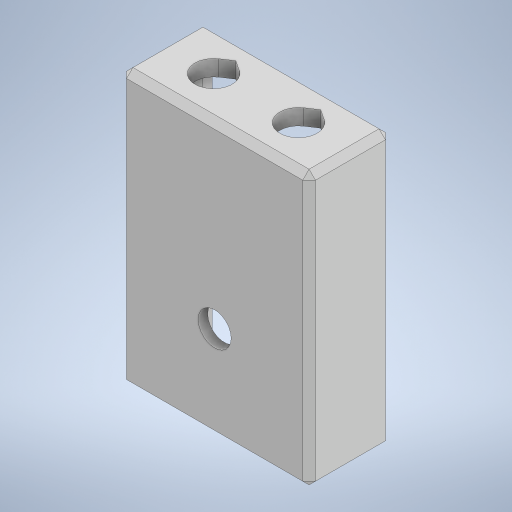
# Autodesk Inventor part: PotiBoxCase
Saved by Autodesk Inventor 2024.3 (Build 283343000, 343)
## iProperties
Created: 2025-03-30
Part Number: PotiBoxCase
Material: Generisch
Document SubType Name: Modeling
Designer: maxho
Density: 1 g/cm^3
Appearance: Vorgabe
Author: maxho
## iProperties of the stored document PotiBoxCase_3D-Druck.ipt
Created: 2025-03-30
Part Number: PotiBoxCase_3D-Druck
Material: Generisch
Document SubType Name: Modeling
Designer: maxho
Density: 1 g/cm^3
Appearance: Vorgabe
Author: maxho
Autodesk Inventor part; units mm, degrees
ref_plane "YZ Plane" through (0, 0, 0) normal (1, 0, 0) x (0, 1, 0)
ref_plane "XZ Plane" through (0, 0, 0) normal (0, 1, 0) x (-1, 0, 0)
ref_plane "XY Plane" through (0, 0, 0) normal (0, 0, 1) x (1, 0, 0)
sketch "Skizze1" plane through (0, 0, 0) normal (0, 1, 0) x (-1, 0, 0)
  line L0 (-29.7, -43) -> (29.7, -43)
  line L1 (29.7, -43) -> (29.7, 43)
  line L2 (29.7, 43) -> (-29.7, 43)
  line L3 (-29.7, 43) -> (-29.7, -43)
  line L4 (-29.7, -43) -> (29.7, 43) construction
  line L5 (29.7, -43) -> (-29.7, 43) construction
  point P0 (0, 0)
  dimension "d2" = 59.4
  dimension "d3" = 86
  constraints: 12 end point, 2 midpoint, 2 parallel, 1 horizontal, 1 perpendicular
  measures "d2" distance of L1.end L2.end
  measures "d3" distance of L0.end L1.end
extrude "Extrusion1" add sketch "Skizze1" along normal blind 26
shell "Wandung1" thickness 3 removed faces 1 at (-9.9, 26, -14.3333)
sketch "Skizze2" plane through (-29.7, 0, 43) normal (0, 0, 1) x (1, 0, 0)
  line L0 (0, 0) -> (59.4, 0) construction
  line L1 (59.4, 0) -> (59.4, 26) construction
  line L2 (0, 26) -> (59.4, 26) construction
  line L3 (0, 0) -> (0, 26) construction
  line L4 (3, 3) -> (56.4, 3) construction
  line L5 (3, 3) -> (3, 26) construction
  line L6 (56.4, 26) -> (3, 26) construction
  line L7 (56.4, 3) -> (56.4, 26) construction
  circle A0 centre (16.35, 13) radius 5.85
  circle A1 centre (43.05, 13) radius 5.85
  line L8 (3, 23) -> (56.4, 23) construction
  line L9 (3, 23) -> (29.7, 3) construction
  line L10 (29.7, 3) -> (56.4, 23) construction
  line L11 (19.5626, 17.8889) -> (16.35, 20)
  line L12 (16.35, 20) -> (13.1374, 17.8889)
  line L13 (46.2626, 17.8889) -> (43.05, 20)
  line L14 (43.05, 20) -> (39.8374, 17.8889)
  point P0 (29.7, 0)
  dimension "d5" = 11.7
  dimension "d19" = 3
  dimension "d20" = 7
  constraints: 14 end point, 4 point on circle, 4 tangent, 3 midpoint, 2 centre point, 2 point on line, 2 vertical alignment, 1 equal radius, 1 horizontal alignment, 1 perpendicular
  measures "d5" diameter of A0
  measures "d19" distance between parallel lines of L2 L8
  measures "d20" distance of A0.centre L11.end
extrude "Extrusion2" cut sketch "Skizze2" against normal up to surface (3 mm away)
sketch "Skizze3" plane through (0, 0, 0) normal (0, -1, 0) x (1, 0, 0)
  line L0 (-29.7, -43) -> (-29.7, 43) construction
  line L1 (29.7, -43) -> (-29.7, -43) construction
  line L2 (29.7, 43) -> (29.7, -43) construction
  line L3 (-29.7, 43) -> (29.7, 43) construction
  line L4 (-26.7, -40) -> (-26.7, 40) construction
  line L5 (-26.7, 40) -> (26.7, 40) construction
  line L6 (26.7, 40) -> (26.7, -40) construction
  line L7 (26.7, -40) -> (-26.7, -40) construction
  circle A0 centre (0, -13.3333) radius 5.205
  line L8 (0, -40) -> (0, -13.3333) construction
  line L9 (0, -13.3333) -> (0, 13.3333) construction
  line L10 (0, 13.3333) -> (0, 40) construction
  point P0 (0, 0)
  dimension "d8" = 10.41
  constraints: 6 end point, 2 collinear, 2 midpoint, 1 centre point, 1 point on line, 1 vertical
  measures "d8" diameter of A0
extrude "Extrusion3" cut sketch "Skizze3" against normal through all
sketch "Skizze4" plane through (29.7, 0, -43) normal (0, 0, -1) x (-1, 0, 0)
  line L0 (0, 0) -> (59.4, 0) construction
  line L1 (59.4, 0) -> (59.4, 26) construction
  line L2 (0, 26) -> (59.4, 26) construction
  line L3 (0, 0) -> (0, 26) construction
  line L4 (3, 3) -> (56.4, 3) construction
  line L5 (24.495, 3) -> (34.905, 3) construction
  line L6 (56.4, 3) -> (3, 3) construction
  line L7 (3, 3) -> (56.4, 3) construction
  line L8 (56.4, 3) -> (56.4, 26) construction
  line L9 (3, 3) -> (3, 26) construction
  line L10 (56.4, 26) -> (57.6426, 23) construction
  line L11 (57.6426, 23) -> (1.7574, 23) construction
  line L12 (1.7574, 23) -> (3, 26) construction
  line L13 (56.5082, 26) -> (57.7923, 22.9)
  line L14 (57.7923, 22.9) -> (1.6077, 22.9)
  line L15 (1.6077, 22.9) -> (2.8918, 26)
  line L16 (2.8918, 26) -> (56.5082, 26)
  line L17 (59.4, 26) -> (0, 26) projected
  point P0 (29.7, 0)
  point P1 (29.7, 26)
  point P2 (29.7, 23)
  point P3 (29.7, 26)
  dimension "d11" = 3
  dimension "d12" = 22.5
  dimension "d13" = 0.1
  constraints: 14 end point, 4 midpoint, 1 collinear, 1 horizontal, 1 vertical alignment, 2 other
  measures "d11" distance between parallel lines of L2 L11
  measures "d12" angle of L10 L8
  measures "d13" distance between parallel lines of L10 L13
extrude "Extrusion4" cut sketch "Skizze4" against normal up to surface (83 mm away)
chamfer "Fasen1" distance 2 angle 45 13 edges at (-29.7, 13, -43) (-29.7, 0, 0) (0, 0, -43) (29.7, 13, -43) (29.7, 0, 0) (0, 0, 43) (-29.7, 13, 43) (29.7, 13, 43) (-29.7, 26, 0) (0, 26, 43) (29.7, 26, 0) (28.2541, 26, -43) (-28.2541, 26, -43)
sketch "Skizze5" plane through (26.7, 3, 40) normal (0, 0, -1) x (-1, 0, 0)
  line L0 (0, 0) -> (0, 19.9) projected
  line L1 (53.4, 0) -> (0, 0) projected
  line L2 (53.4, 0) -> (53.4, 19.9) projected
  line L3 (53.4, 19.9) -> (54.7923, 19.9) projected
  line L4 (54.7923, 19.9) -> (53.5082, 23) projected
  line L5 (-0.1082, 23) -> (53.5082, 23) projected
  line L6 (-0.1082, 23) -> (-1.3923, 19.9) projected
  line L7 (-1.3923, 19.9) -> (0, 19.9) projected
  arc A0 (10.1374, 14.8889) -> (16.5626, 14.8889) centre (13.35, 10) ccw projected
  line L8 (10.1374, 14.8889) -> (13.35, 17) projected
  line L9 (13.35, 17) -> (16.5626, 14.8889) projected
  line L10 (40.05, 17) -> (43.2626, 14.8889) projected
  arc A1 (36.8374, 14.8889) -> (43.2626, 14.8889) centre (40.05, 10) ccw projected
  line L11 (36.8374, 14.8889) -> (40.05, 17) projected
  line L12 (0, 19.9) -> (53.4, 19.9)
  point P0 (26.7, -3)
  constraints: 2 end point, 1 horizontal
extrude "Extrusion5" add sketch "Skizze5" along normal blind 2 contours L0 L12 L2 L1
sketch "Skizze6" plane through (-26.7, 3, -40) normal (0, 1, 0) x (1, 0, 0)
  line L0 (18.1388, -45.7075) -> (30.6952, -45.7075) construction
  line L1 (30.6952, -45.7075) -> (30.6952, -51.3198) construction
  line L2 (30.6952, -51.3198) -> (18.1388, -51.3198) construction
  line L3 (18.1388, -51.3198) -> (18.1388, -45.7075) construction
  line L4 (20.9099, -49.2784) -> (18.5983, -49.2784)
  line L5 (18.5983, -49.2784) -> (18.5983, -48.6686)
  line L6 (18.5983, -48.6686) -> (19.3357, -48.6686)
  line L7 (19.3357, -48.6686) -> (19.3357, -46.8165)
  line L8 (19.3357, -46.8165) -> (18.5983, -46.8165)
  line L9 (18.5983, -46.8165) -> (18.5983, -46.2464)
  spline S0 degree 2 poles (18.5983, -46.2464) (18.76, -46.2464) (19.0805, -46.2038) (19.1769, -46.1584) knots 0 0 0 1 2 2 2
  spline S1 degree 2 poles (19.1769, -46.1584) (19.2875, -46.1017) (19.4123, -45.9117) (19.4237, -45.7699) knots 0 0 0 1 2 2 2
  line L10 (19.4237, -45.7699) -> (20.1895, -45.7699)
  line L11 (20.1895, -45.7699) -> (20.1895, -48.6686)
  line L12 (20.1895, -48.6686) -> (20.9099, -48.6686)
  line L13 (20.9099, -48.6686) -> (20.9099, -49.2784)
  line L14 (22.3706, -49.2784) -> (21.5395, -49.2784)
  line L15 (21.5395, -49.2784) -> (21.5395, -48.3537)
  line L16 (21.5395, -48.3537) -> (22.3706, -48.3537)
  line L17 (22.3706, -48.3537) -> (22.3706, -49.2784)
  line L18 (25.4792, -49.2784) -> (23.1676, -49.2784)
  line L19 (23.1676, -49.2784) -> (23.1676, -48.6686)
  line L20 (23.1676, -48.6686) -> (23.905, -48.6686)
  line L21 (23.905, -48.6686) -> (23.905, -46.8165)
  line L22 (23.905, -46.8165) -> (23.1676, -46.8165)
  line L23 (23.1676, -46.8165) -> (23.1676, -46.2464)
  spline S2 degree 2 poles (23.1676, -46.2464) (23.3292, -46.2464) (23.6497, -46.2038) (23.7462, -46.1584) knots 0 0 0 1 2 2 2
  spline S3 degree 2 poles (23.7462, -46.1584) (23.8568, -46.1017) (23.9816, -45.9117) (23.9929, -45.7699) knots 0 0 0 1 2 2 2
  line L24 (23.9929, -45.7699) -> (24.7587, -45.7699)
  line L25 (24.7587, -45.7699) -> (24.7587, -48.6686)
  line L26 (24.7587, -48.6686) -> (25.4792, -48.6686)
  line L27 (25.4792, -48.6686) -> (25.4792, -49.2784)
  line L28 (26.9399, -49.2784) -> (26.1088, -49.2784)
  line L29 (26.1088, -49.2784) -> (26.1088, -48.3537)
  line L30 (26.1088, -48.3537) -> (26.9399, -48.3537)
  line L31 (26.9399, -48.3537) -> (26.9399, -49.2784)
  spline S4 degree 2 poles (30.1591, -47.5284) (30.1591, -47.9822) (30.0144, -48.6629) (29.8527, -48.8926) knots 0 0 0 1 2 2 2
  spline S5 degree 2 poles (29.8527, -48.8926) (29.6939, -49.1195) (29.1805, -49.3521) (28.8118, -49.3521) knots 0 0 0 1 2 2 2
  spline S6 degree 2 poles (28.8118, -49.3521) (28.4403, -49.3521) (27.9297, -49.1195) (27.7681, -48.887) knots 0 0 0 1 2 2 2
  spline S7 degree 2 poles (27.7681, -48.887) (27.6064, -48.6572) (27.4617, -47.9822) (27.4617, -47.5284) knots 0 0 0 1 2 2 2
  spline S8 degree 2 poles (27.4617, -47.5284) (27.4617, -47.0632) (27.6064, -46.4052) (27.7709, -46.1669) knots 0 0 0 1 2 2 2
  spline S9 degree 2 poles (27.7709, -46.1669) (27.9354, -45.9344) (28.4544, -45.7075) (28.8118, -45.7075) knots 0 0 0 1 2 2 2
  spline S10 degree 2 poles (28.8118, -45.7075) (29.189, -45.7075) (29.6939, -45.9457) (29.8556, -46.1811) knots 0 0 0 1 2 2 2
  spline S11 degree 2 poles (29.8556, -46.1811) (30.0144, -46.4109) (30.1591, -47.0887) (30.1591, -47.5284) knots 0 0 0 1 2 2 2
  spline S12 degree 2 poles (29.277, -47.5284) (29.277, -46.8789) (29.0643, -46.3541) (28.8118, -46.3541) knots 0 0 0 1 2 2 2
  spline S13 degree 2 poles (28.8118, -46.3541) (28.5594, -46.3541) (28.3438, -46.8789) (28.3438, -47.5312) knots 0 0 0 1 2 2 2
  spline S14 degree 2 poles (28.3438, -47.5312) (28.3438, -48.1722) (28.5594, -48.7054) (28.8118, -48.7054) knots 0 0 0 1 2 2 2
  spline S15 degree 2 poles (28.8118, -48.7054) (29.0614, -48.7054) (29.277, -48.1722) (29.277, -47.5284) knots 0 0 0 1 2 2 2
  point P0 (26.7, -40)
  constraints: 2 other
emboss "Prägen1" sketch "Skizze6" operation cut depth 0.5 direction (0, -1, 0)
equation "\"d2\" = PotiBoxInnerWidth + 2 * PotiBoxThickness"
equation "\"d3\" = PotiBoxInnerLength + 2 * PotiBoxThickness"
equation "\"d0\" = PotiBoxInnerHeight + 2 * PotiBoxThickness"
equation "\"d4\" = PotiBoxThickness"
equation "\"d5\" = ConnectorDiameter"
equation "\"d19\" = PotiBoxThickness"
equation "\"d8\" = PotiDiameter"
equation "\"d11\" = PotiBoxThickness"
equation "\"d13\" = Clearance"
equation "\"PotiBoxInnerWidth\" = 53.4"
equation "\"PotiBoxThickness\" = 3"
equation "\"PotiBoxInnerLength\" = 80"
equation "\"PotiBoxInnerHeight\" = 20"
equation "\"ConnectorDiameter\" = 11.7"
equation "\"PotiDiameter\" = 10.41"
equation "\"Clearance\" = 0.1"
